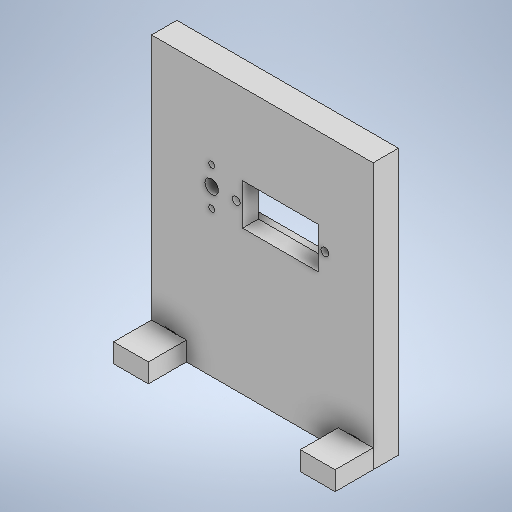
# Autodesk Inventor part: Turm_Servo
Saved by Autodesk Inventor 2025 (Build 290162000, 162)
## iProperties
Created: 2026-07-08
Part Number: Turm_Servo
Material: Generisch
Document SubType Name: Modeling
Designer: wavid
Mass: 45.2671 g
Surface Area: 155.902 cm^2
Volume: 45.2671 cm^3
Density: 1 g/cm^3
Appearance: Vorgabe
Author: wavid
Autodesk Inventor part; units mm, degrees
ref_plane "YZ Plane" through (0, 0, 0) normal (1, 0, 0) x (0, 1, 0)
ref_plane "XY Plane" through (0, 0, 0) normal (0, 0, 1) x (1, 0, 0)
sketch "Skizze1" plane through (0, 0, 0) normal (0, 0, 1) x (1, 0, 0)
  line L0 (-35, 0) -> (35, 0)
  line L1 (35, 0) -> (35, 8)
  line L2 (35, 8) -> (-35, 8)
  line L3 (-35, 8) -> (-35, 0)
  constraints: 8 end point, 2 parallel, 1 horizontal, 1 perpendicular
extrude "Extrusion1" add sketch "Skizze1" along normal blind 84
sketch "Skizze2" plane through (0, 0, 0) normal (0, 0, 1) x (1, 0, 0)
  line L0 (-35, -12) -> (-24, -12)
  line L1 (-24, -12) -> (-24, 0)
  line L2 (-24, 0) -> (-35, 0)
  line L3 (-35, 0) -> (-35, -12)
  constraints: 8 end point, 2 parallel, 1 horizontal, 1 perpendicular
extrude "Extrusion2" add sketch "Skizze2" along normal blind 6 separate body
sketch "Skizze3" plane through (0, 0, 0) normal (0, 0, 1) x (1, 0, 0)
  line L0 (24, -12) -> (35, -12)
  line L1 (35, -12) -> (35, 0)
  line L2 (35, 0) -> (24, 0)
  line L3 (24, 0) -> (24, -12)
  constraints: 8 end point, 2 parallel, 1 horizontal, 1 perpendicular
extrude "Extrusion3" add sketch "Skizze3" along normal blind 6 separate body
sketch "Skizze4" plane through (0, 0, 0) normal (0, 0, 1) x (1, 0, 0)
  circle A0 centre (-29, 0) radius 1.7
  constraints: 1 centre point
extrude "Extrusion4" cut sketch "Skizze4" along normal blind 6.2 bodies 1
sketch "Skizze5" plane through (0, 0, 0) normal (0, 0, 1) x (1, 0, 0)
  circle A0 centre (29, 0) radius 1.7
  constraints: 1 centre point
extrude "Extrusion5" cut sketch "Skizze5" along normal blind 6.2 bodies 1
sketch "Skizze6" plane through (0, 0, 0) normal (0, 1, 0) x (-1, 0, 0)
  line L0 (-17.75, 45.5) -> (6.25, 45.5)
  line L1 (6.25, 45.5) -> (6.25, 58.5)
  line L2 (6.25, 58.5) -> (-17.75, 58.5)
  line L3 (-17.75, 58.5) -> (-17.75, 45.5)
  constraints: 8 end point, 2 parallel, 1 horizontal, 1 perpendicular
extrude "Extrusion6" cut sketch "Skizze6" along normal blind 8.2 bodies 1
sketch "Skizze7" plane through (0, 0, 0) normal (0, 1, 0) x (-1, 0, 0)
  circle A0 centre (-19.75, 52) radius 1.25
  constraints: 1 centre point
extrude "Extrusion7" cut sketch "Skizze7" along normal blind 8.2 bodies 1
sketch "Skizze8" plane through (0, 0, 0) normal (0, 1, 0) x (-1, 0, 0)
  circle A0 centre (8.25, 52) radius 1.25
  constraints: 1 centre point
extrude "Extrusion8" cut sketch "Skizze8" along normal blind 8.2 bodies 1
sketch "Skizze9" plane through (0, 0, 0) normal (0, 1, 0) x (-1, 0, 0)
  circle A0 centre (16, 52) radius 2.15
  constraints: 1 centre point
extrude "Extrusion9" cut sketch "Skizze9" along normal blind 8.2 bodies 1
sketch "Skizze10" plane through (0, 0, 0) normal (0, 1, 0) x (-1, 0, 0)
  circle A0 centre (16, 46) radius 0.95
  constraints: 1 centre point
extrude "Extrusion10" cut sketch "Skizze10" along normal blind 8.2 bodies 1
sketch "Skizze11" plane through (0, 0, 0) normal (0, 1, 0) x (-1, 0, 0)
  circle A0 centre (16, 58) radius 0.95
  constraints: 1 centre point
extrude "Extrusion11" cut sketch "Skizze11" along normal blind 8.2 bodies 1
ref_plane "Arbeitsebene1" through (0, 5, 0) normal (0, 1, 0) x (-1, 0, 0)
sketch "Skizze12" plane through (0, 5, 0) normal (0, 1, 0) x (-1, 0, 0)
  line L0 (-22.75, 44.5) -> (11.25, 44.5)
  line L1 (11.25, 44.5) -> (11.25, 59.5)
  line L2 (11.25, 59.5) -> (-22.75, 59.5)
  line L3 (-22.75, 59.5) -> (-22.75, 44.5)
  constraints: 8 end point, 2 parallel, 1 horizontal, 1 perpendicular
extrude "Extrusion12" cut sketch "Skizze12" along normal blind 3.2 bodies 1
